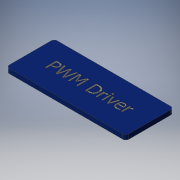
# Autodesk Inventor part: PWM Driver
Saved by Autodesk Inventor 2016 (Build 200138000, 138)
## iProperties
Created: 2015-10-05
Part Number: PWM Driver
Material: Generic
Document SubType Name: Modeling
Designer: powasar16
Density: 1 g/cm^3
Appearance: Default
Author: powasar16
Autodesk Inventor part; units mm, degrees
note: some values were not read from the file. Chosen so that the rebuilt part matches the saved one: direction of "Emboss1".
ref_plane "YZ Plane" through (0, 0, 0) normal (1, 0, 0) x (0, 1, 0)
ref_plane "XZ Plane" through (0, 0, 0) normal (0, 1, 0) x (-1, 0, 0)
ref_plane "XY Plane" through (0, 0, 0) normal (0, 0, 1) x (1, 0, 0)
sketch "Sketch1" plane through (0, 0, 0) normal (0, 1, 0) x (-1, 0, 0)
  line L0 (-1.5875, 0) -> (-61.9125, 0)
  line L1 (-63.5, -1.5875) -> (-63.5, -23.8125)
  line L2 (-61.9125, -25.4) -> (-1.5875, -25.4)
  line L3 (0, -23.8125) -> (0, -1.5875)
  arc A0 (0, -1.5875) -> (-1.5875, 0) centre (-1.5875, -1.5875) ccw
  line L4 (-31.75, -25.4) -> (-31.75, 0) construction
  line L5 (0, -12.7) -> (-63.5, -12.7) construction
  arc A1 (-61.9125, 0) -> (-63.5, -1.5875) centre (-61.9125, -1.5875) ccw
  arc A2 (-1.5875, -25.4) -> (0, -23.8125) centre (-1.5875, -23.8125) ccw
  arc A3 (-63.5, -23.8125) -> (-61.9125, -25.4) centre (-61.9125, -23.8125) ccw
  point P0 (0, 0)
  dimension "d2" = 3.175
  dimension "d5" = 60.325
  dimension "d6" = 60.325
  dimension "d7" = 22.225
  constraints: 12 end point, 9 symmetric about line, 8 point on circle, 4 centre point, 4 midpoint, 2 horizontal, 2 parallel, 2 tangent, 1 perpendicular, 1 vertical, 3 other
  measures "d2" diameter of A0
  measures "d5" distance of A3.centre A2.centre
  measures "d6" distance of A1.centre A0.centre
  measures "d7" distance of A3.centre A1.centre
extrude "Extrusion1" add sketch "Sketch1" along normal blind 2.54
sketch "Sketch2" plane through (0, 2.54, 0) normal (0, 1, 0) x (1, 0, 0)
  line L0 (61.9125, 25.4) -> (1.5875, 25.4) projected
  arc A0 (1.5875, 25.4) -> (0, 23.8125) centre (1.5875, 23.8125) ccw projected
  line L1 (0, 23.8125) -> (0, 1.5875) projected
  arc A1 (0, 1.5875) -> (1.5875, 0) centre (1.5875, 1.5875) ccw projected
  line L2 (1.5875, 0) -> (61.9125, 0) projected
  arc A2 (61.9125, 0) -> (63.5, 1.5875) centre (61.9125, 1.5875) ccw projected
  line L3 (63.5, 1.5875) -> (63.5, 23.8125) projected
  arc A3 (63.5, 23.8125) -> (61.9125, 25.4) centre (61.9125, 23.8125) ccw projected
  line L4 (9.9229, 16.0627) -> (63.8786, 16.0627) construction
  line L5 (63.8786, 16.0627) -> (63.8786, -1.5505) construction
  line L6 (63.8786, -1.5505) -> (9.9229, -1.5505) construction
  line L7 (9.9229, -1.5505) -> (9.9229, 16.0627) construction
  spline S0 degree 2 poles (14.3936, 14.1855) (14.3936, 13.7903) (14.112, 13.0789) (13.8601, 12.8319) knots 0 0 0 1 2 2 2
  spline S1 degree 2 poles (13.8601, 12.8319) (13.5439, 12.5207) (12.6893, 12.1996) (12.0372, 12.1996) knots 0 0 0 1 2 2 2
  line L8 (12.0372, 12.1996) -> (11.3506, 12.1996)
  line L9 (11.3506, 12.1996) -> (11.3506, 9.9272)
  line L10 (11.3506, 9.9272) -> (10.5404, 9.9272)
  line L11 (10.5404, 9.9272) -> (10.5404, 16.0232)
  line L12 (10.5404, 16.0232) -> (12.0718, 16.0232)
  spline S2 degree 2 poles (12.0718, 16.0232) (12.6152, 16.0232) (13.376, 15.8453) (13.6674, 15.6428) knots 0 0 0 1 2 2 2
  spline S3 degree 2 poles (13.6674, 15.6428) (14.0083, 15.4106) (14.3936, 14.6943) (14.3936, 14.1855) knots 0 0 0 1 2 2 2
  spline S4 degree 2 poles (13.5489, 14.1608) (13.5489, 14.4769) (13.3315, 14.9413) (13.1092, 15.0895) knots 0 0 0 1 2 2 2
  spline S5 degree 2 poles (13.1092, 15.0895) (12.9166, 15.2179) (12.4028, 15.3217) (12.0224, 15.3217) knots 0 0 0 1 2 2 2
  line L13 (12.0224, 15.3217) -> (11.3506, 15.3217)
  line L14 (11.3506, 15.3217) -> (11.3506, 12.8912)
  line L15 (11.3506, 12.8912) -> (11.9038, 12.8912)
  spline S6 degree 2 poles (11.9038, 12.8912) (12.3979, 12.8912) (13.0055, 13.0493) (13.2031, 13.2567) knots 0 0 0 1 2 2 2
  spline S7 degree 2 poles (13.2031, 13.2567) (13.3859, 13.4395) (13.5489, 13.8693) (13.5489, 14.1608) knots 0 0 0 1 2 2 2
  line L16 (21.9963, 16.0232) -> (20.4649, 9.9272)
  line L17 (20.4649, 9.9272) -> (19.556, 9.9272)
  line L18 (19.556, 9.9272) -> (18.316, 14.9858)
  line L19 (18.316, 14.9858) -> (17.1106, 9.9272)
  line L20 (17.1106, 9.9272) -> (16.2116, 9.9272)
  line L21 (16.2116, 9.9272) -> (14.6554, 16.0232)
  line L22 (14.6554, 16.0232) -> (15.4903, 16.0232)
  line L23 (15.4903, 16.0232) -> (16.7154, 10.9695)
  line L24 (16.7154, 10.9695) -> (17.9307, 16.0232)
  line L25 (17.9307, 16.0232) -> (18.7557, 16.0232)
  line L26 (18.7557, 16.0232) -> (19.9808, 10.9102)
  line L27 (19.9808, 10.9102) -> (21.201, 16.0232)
  line L28 (21.201, 16.0232) -> (21.9963, 16.0232)
  line L29 (27.9491, 9.9272) -> (27.1389, 9.9272)
  line L30 (27.1389, 9.9272) -> (27.1389, 15.1784)
  line L31 (27.1389, 15.1784) -> (25.5482, 11.6068)
  line L32 (25.5482, 11.6068) -> (25.0542, 11.6068)
  line L33 (25.0542, 11.6068) -> (23.4783, 15.1784)
  line L34 (23.4783, 15.1784) -> (23.4783, 9.9272)
  line L35 (23.4783, 9.9272) -> (22.7225, 9.9272)
  line L36 (22.7225, 9.9272) -> (22.7225, 16.0232)
  line L37 (22.7225, 16.0232) -> (23.8291, 16.0232)
  line L38 (23.8291, 16.0232) -> (25.3506, 12.6294)
  line L39 (25.3506, 12.6294) -> (26.8227, 16.0232)
  line L40 (26.8227, 16.0232) -> (27.9491, 16.0232)
  line L41 (27.9491, 16.0232) -> (27.9491, 9.9272)
  spline S8 degree 2 poles (36.6089, 12.9702) (36.6089, 12.1354) (35.9322, 10.7917) (35.3641, 10.4162) knots 0 0 0 1 2 2 2
  spline S9 degree 2 poles (35.3641, 10.4162) (34.8997, 10.1248) (33.9463, 9.9272) (33.2053, 9.9272) knots 0 0 0 1 2 2 2
  line L42 (33.2053, 9.9272) -> (31.8023, 9.9272)
  line L43 (31.8023, 9.9272) -> (31.8023, 16.0232)
  line L44 (31.8023, 16.0232) -> (33.1904, 16.0232)
  spline S10 degree 2 poles (33.1904, 16.0232) (34.05, 16.0232) (35.0281, 15.7663) (35.3739, 15.539) knots 0 0 0 1 2 2 2
  spline S11 degree 2 poles (35.3739, 15.539) (35.9618, 15.1488) (36.6089, 13.8594) (36.6089, 12.9702) knots 0 0 0 1 2 2 2
  spline S12 degree 2 poles (35.7642, 12.9801) (35.7642, 13.6816) (35.2998, 14.6745) (34.8404, 14.9561) knots 0 0 0 1 2 2 2
  spline S13 degree 2 poles (34.8404, 14.9561) (34.5144, 15.1488) (33.7783, 15.3217) (33.23, 15.3217) knots 0 0 0 1 2 2 2
  line L45 (33.23, 15.3217) -> (32.6125, 15.3217)
  line L46 (32.6125, 15.3217) -> (32.6125, 10.6287)
  line L47 (32.6125, 10.6287) -> (33.23, 10.6287)
  spline S14 degree 2 poles (33.23, 10.6287) (33.7684, 10.6287) (34.5835, 10.8016) (34.9145, 11.0337) knots 0 0 0 1 2 2 2
  spline S15 degree 2 poles (34.9145, 11.0337) (35.3394, 11.3203) (35.7642, 12.2687) (35.7642, 12.9801) knots 0 0 0 1 2 2 2
  line L48 (39.8546, 13.6767) -> (39.815, 13.6767)
  spline S16 degree 2 poles (39.815, 13.6767) (39.7261, 13.7014) (39.5334, 13.7112) (39.4001, 13.7112) knots 0 0 0 1 2 2 2
  spline S17 degree 2 poles (39.4001, 13.7112) (39.0888, 13.7112) (38.4763, 13.4395) (38.1996, 13.1728) knots 0 0 0 1 2 2 2
  line L49 (38.1996, 13.1728) -> (38.1996, 9.9272)
  line L50 (38.1996, 9.9272) -> (37.429, 9.9272)
  line L51 (37.429, 9.9272) -> (37.429, 14.5016)
  line L52 (37.429, 14.5016) -> (38.1996, 14.5016)
  line L53 (38.1996, 14.5016) -> (38.1996, 13.8199)
  spline S18 degree 2 poles (38.1996, 13.8199) (38.6195, 14.1954) (39.2469, 14.5016) (39.5433, 14.5016) knots 0 0 0 1 2 2 2
  spline S19 degree 2 poles (39.5433, 14.5016) (39.6619, 14.5016) (39.7805, 14.4918) (39.8546, 14.4769) knots 0 0 0 1 2 2 2
  line L54 (39.8546, 14.4769) -> (39.8546, 13.6767)
  line L55 (41.2378, 9.9272) -> (40.4671, 9.9272)
  line L56 (40.4671, 9.9272) -> (40.4671, 14.5016)
  line L57 (40.4671, 14.5016) -> (41.2378, 14.5016)
  line L58 (41.2378, 14.5016) -> (41.2378, 9.9272)
  line L59 (41.2921, 15.2624) -> (40.4177, 15.2624)
  line L60 (40.4177, 15.2624) -> (40.4177, 16.0627)
  line L61 (40.4177, 16.0627) -> (41.2921, 16.0627)
  line L62 (41.2921, 16.0627) -> (41.2921, 15.2624)
  line L63 (45.9604, 14.5016) -> (44.2364, 9.9272)
  line L64 (44.2364, 9.9272) -> (43.5448, 9.9272)
  line L65 (43.5448, 9.9272) -> (41.8355, 14.5016)
  line L66 (41.8355, 14.5016) -> (42.6704, 14.5016)
  line L67 (42.6704, 14.5016) -> (43.9202, 10.9794)
  line L68 (43.9202, 10.9794) -> (45.1601, 14.5016)
  line L69 (45.1601, 14.5016) -> (45.9604, 14.5016)
  spline S20 degree 2 poles (48.5292, 9.8234) (47.4326, 9.8234) (46.2272, 11.0535) (46.2272, 12.1897) knots 0 0 0 1 2 2 2
  spline S21 degree 2 poles (46.2272, 12.1897) (46.2272, 13.3062) (47.398, 14.6301) (48.3415, 14.6301) knots 0 0 0 1 2 2 2
  spline S22 degree 2 poles (48.3415, 14.6301) (48.7664, 14.6301) (49.4234, 14.3831) (49.6655, 14.1213) knots 0 0 0 1 2 2 2
  spline S23 degree 2 poles (49.6655, 14.1213) (49.9125, 13.8594) (50.1743, 13.1036) (50.1743, 12.5553) knots 0 0 0 1 2 2 2
  line L70 (50.1743, 12.5553) -> (50.1743, 12.1354)
  line L71 (50.1743, 12.1354) -> (47.0077, 12.1354)
  spline S24 degree 2 poles (47.0077, 12.1354) (47.0077, 11.34) (47.808, 10.4953) (48.5194, 10.4953) knots 0 0 0 1 2 2 2
  spline S25 degree 2 poles (48.5194, 10.4953) (48.7713, 10.4953) (49.2604, 10.6089) (49.458, 10.6978) knots 0 0 0 1 2 2 2
  spline S26 degree 2 poles (49.458, 10.6978) (49.6655, 10.7966) (49.952, 10.9695) (50.0458, 11.0486) knots 0 0 0 1 2 2 2
  line L72 (50.0458, 11.0486) -> (50.0903, 11.0486)
  line L73 (50.0903, 11.0486) -> (50.0903, 10.2087)
  spline S27 degree 2 poles (50.0903, 10.2087) (49.9569, 10.1544) (49.5518, 9.9963) (49.3938, 9.9519) knots 0 0 0 1 2 2 2
  spline S28 degree 2 poles (49.3938, 9.9519) (49.1715, 9.8876) (48.8059, 9.8234) (48.5292, 9.8234) knots 0 0 0 1 2 2 2
  spline S29 degree 2 poles (49.4234, 12.7232) (49.4135, 13.0344) (49.2851, 13.4889) (49.1616, 13.6421) knots 0 0 0 1 2 2 2
  spline S30 degree 2 poles (49.1616, 13.6421) (49.0282, 13.815) (48.6083, 13.9978) (48.2971, 13.9978) knots 0 0 0 1 2 2 2
  spline S31 degree 2 poles (48.2971, 13.9978) (47.9908, 13.9978) (47.561, 13.815) (47.3832, 13.6371) knots 0 0 0 1 2 2 2
  spline S32 degree 2 poles (47.3832, 13.6371) (47.2103, 13.4544) (47.0324, 13.0147) (47.0077, 12.7232) knots 0 0 0 1 2 2 2
  line L74 (47.0077, 12.7232) -> (49.4234, 12.7232)
  line L75 (53.3804, 13.6767) -> (53.3408, 13.6767)
  spline S33 degree 2 poles (53.3408, 13.6767) (53.2519, 13.7014) (53.0593, 13.7112) (52.9259, 13.7112) knots 0 0 0 1 2 2 2
  spline S34 degree 2 poles (52.9259, 13.7112) (52.6147, 13.7112) (52.0021, 13.4395) (51.7254, 13.1728) knots 0 0 0 1 2 2 2
  line L76 (51.7254, 13.1728) -> (51.7254, 9.9272)
  line L77 (51.7254, 9.9272) -> (50.9548, 9.9272)
  line L78 (50.9548, 9.9272) -> (50.9548, 14.5016)
  line L79 (50.9548, 14.5016) -> (51.7254, 14.5016)
  line L80 (51.7254, 14.5016) -> (51.7254, 13.8199)
  spline S35 degree 2 poles (51.7254, 13.8199) (52.1454, 14.1954) (52.7727, 14.5016) (53.0691, 14.5016) knots 0 0 0 1 2 2 2
  spline S36 degree 2 poles (53.0691, 14.5016) (53.1877, 14.5016) (53.3063, 14.4918) (53.3804, 14.4769) knots 0 0 0 1 2 2 2
  line L81 (53.3804, 14.4769) -> (53.3804, 13.6767)
  point P0 (0, 0)
  constraints: 2 other
emboss "Emboss1" sketch "Sketch2" operation cut depth 1.27 direction (0, -1, 0) contours S0 S1 L8 L9 L10 L11 L12 S2 S3 | L16 L17 L18 L19 L20 L21 L22 L23 L24 L25 L26 L27 L28 | L29 L30 L31 L32 L33 L34 L35 L36 L37 L38 L39 L40 L41 | S8 S9 L42 L43 L44 S10 S11 | L48 S16 S17 L49 L50 L51 L52 L53 S18 S19 L54 | L55 L56 L57 L58 | L59 L60 L61 L62 | L63 L64 L65 L66 L67 L68 L69 | S20 S21 S22 S23 L70 L71 S24 S25 S26 L72 L73 S27 S28 | L75 S33 S34 L76 L77 L78 L79 L80 S35 S36 L81
body "Solid1"
